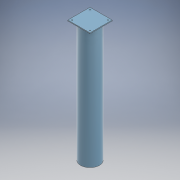
# Autodesk Inventor part: RaAxis
Saved by Autodesk Inventor 2022 (Build 260153000, 153)
## iProperties
Created: 2021-05-01
Part Number: RaAxis
Material: Generic
Document SubType Name: Modeling
Designer: Mick Veldhuis
Density: 1 g/cm^3
Appearance: Default
Author: Mick Veldhuis
Autodesk Inventor part; units mm, degrees
ref_plane "YZ Plane" through (0, 0, 0) normal (1, 0, 0) x (0, 1, 0)
ref_plane "XZ Plane" through (0, 0, 0) normal (0, 1, 0) x (-1, 0, 0)
sketch "Sketch1" plane through (0, 0, 0) normal (0, 1, 0) x (-1, 0, 0)
  circle A0 centre (0, 0) radius 80
  constraints: 1 centre point, 1 coincident
extrude "InBase" add sketch "Sketch1" along normal blind 400
sketch "Sketch2" plane through (0, 400, 0) normal (0, 1, 0) x (1, 0, 0)
  circle A0 centre (0, 0) radius 80
  constraints: 1 centre point, 1 coincident
extrude "AboveBase" add sketch "Sketch2" along normal blind 620
ref_plane "PlateWorkPlane" through (0, 1020, 0) normal (0, 1, 0) x (1, 0, 0)
sketch "Sketch3" plane through (0, 1020, 0) normal (0, 1, 0) x (1, 0, 0)
  line L0 (-94, -94) -> (94, -94)
  line L1 (94, -94) -> (94, 94)
  line L2 (94, 94) -> (-94, 94)
  line L3 (-94, 94) -> (-94, -94)
  line L4 (-94, -94) -> (94, 94) construction
  line L5 (94, -94) -> (-94, 94) construction
  point P0 (0, 0)
  constraints: 12 end point, 2 midpoint, 2 parallel, 1 horizontal, 1 perpendicular
extrude "ConnectorPlate" add sketch "Sketch3" along normal blind 8
sketch "Sketch4" plane through (0, 1020, 0) normal (0, -1, 0) x (1, 0, 0)
  point P0 (0, 0)
  point P1 (-76, -76)
  point P2 (-76, 76)
  point P3 (76, 76)
  point P4 (76, -76)
hole "BoltHoles" at (-76, 1020, 76) at (76, 1020, 76) at (76, 1020, -76) at (-76, 1020, -76) direction (0, 1, 0) diameter 8 end through all
fillet "Fillet1" radius 1 4 edges at (0, 1020, 94) (94, 1020, 0) (-94, 1020, 0) (0, 1020, -94)
body "Solid1"
